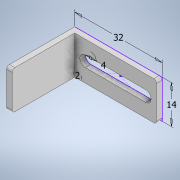
# Autodesk Inventor part: actuator_backbone_fixings_for_measurements
Saved by Autodesk Inventor 2021 (Build 250183000, 183)
## iProperties
Created: 2021-09-01
Part Number: actuator_backbone_fixings_for_measurements
Material: Generic
Document SubType Name: Modeling
Designer: Charlie
Density: 1 g/cm^3
Appearance: Default
Author: Charlie
Autodesk Inventor part; units mm, degrees
ref_plane "YZ Plane" through (0, 0, 0) normal (1, 0, 0) x (0, 1, 0)
ref_plane "XZ Plane" through (0, 0, 0) normal (0, 1, 0) x (-1, 0, 0)
ref_plane "XY Plane" through (0, 0, 0) normal (0, 0, 1) x (1, 0, 0)
sketch "Sketch1" plane through (0, 0, 0) normal (0, 0, 1) x (1, 0, 0)
  line L0 (-14.5, -7) -> (17.5, -7)
  line L1 (17.5, -7) -> (17.5, 7)
  line L2 (17.5, 7) -> (-14.5, 7)
  line L3 (-14.5, 7) -> (-14.5, -7)
  line L4 (-14.5, -7) -> (17.5, 7) construction
  line L5 (17.5, -7) -> (-14.5, 7) construction
  line L6 (-14.5, 7) -> (-12.5, 7)
  line L7 (-12.5, 7) -> (-12.5, -7)
  line L8 (-12.5, -7) -> (-14.5, -7)
  line L9 (-14.5, -7) -> (-14.5, 7)
  line L10 (13.4907, 0) -> (-8.632, 0) construction
  line L11 (13.4907, 2) -> (-8.632, 2)
  line L12 (-8.632, -2) -> (13.4907, -2)
  arc A0 (13.4907, -2) -> (13.4907, 2) centre (13.4907, 0) ccw
  arc A1 (-8.632, 2) -> (-8.632, -2) centre (-8.632, 0) ccw
  point P0 (2.4294, 0)
  dimension "d0" = 32
  dimension "d1" = 14
  dimension "d4" = 2
  dimension "d6" = 4
  constraints: 28 end point, 5 parallel, 4 point on circle, 4 tangent, 3 horizontal, 2 centre point, 2 perpendicular, 1 midpoint, 1 point on line
  measures "d0" distance of L2.end L1.end
  measures "d1" distance of L1.end L0.end
  measures "d4" distance of L7.end L8.end
  measures "d6" diameter of A1
extrude "Extrusion1" add sketch "Sketch1" along normal blind 2
extrude "Extrusion2" add sketch "Sketch1" along normal blind 25 contours L3 L2 L7 L0
fillet "Fillet1" radius 1 4 edges at (17.5, -7, 1) (17.5, 7, 1) (-13.5, 7, 25) (-13.5, -7, 25)
body "Solid1"
